Autodesk Inventor part; units mm, degrees
(part 3 of 5)
sketch "Skizze6" plane through (0, 1, 0) normal (0, 1, 0) x (1, 0, 0)
  line L0 (-132.892, -90.8566) -> (-0.05, -90.8566) projected
  line L1 (-0.05, -90.8566) -> (-0.05, -0.0262) projected
  line L2 (-0.05, -0.0262) -> (-132.892, -0.0262) projected
  line L3 (-132.892, -0.0262) -> (-132.892, -90.8566) projected
  line L4 (-22.1876, -19.3868) -> (-20.5876, -19.3868) projected
  line L5 (-20.5876, -19.3868) -> (-20.5876, -20.0368) projected
  line L6 (-20.5876, -20.0368) -> (-22.1876, -20.0368) projected
  line L7 (-22.1876, -20.0368) -> (-22.1876, -19.3868) projected
  line L8 (-22.1876, -11.4868) -> (-20.5876, -11.4868) projected
  line L9 (-20.5876, -11.4868) -> (-20.5876, -12.1368) projected
  line L10 (-20.5876, -12.1368) -> (-22.1876, -12.1368) projected
  line L11 (-22.1876, -12.1368) -> (-22.1876, -11.4868) projected
  line L12 (-23.0526, -18.3618) -> (-22.2626, -18.3618) projected
  line L13 (-22.2626, -18.3618) -> (-22.2626, -18.7618) projected
  line L14 (-22.2626, -18.7618) -> (-23.0526, -18.7618) projected
  line L15 (-23.0526, -18.7618) -> (-23.0526, -18.3618) projected
  line L16 (-20.5126, -18.3618) -> (-19.7226, -18.3618) projected
  line L17 (-19.7226, -18.3618) -> (-19.7226, -18.7618) projected
  line L18 (-19.7226, -18.7618) -> (-20.5126, -18.7618) projected
  line L19 (-20.5126, -18.7618) -> (-20.5126, -18.3618) projected
  line L20 (-23.0526, -17.5618) -> (-22.2626, -17.5618) projected
  line L21 (-22.2626, -17.5618) -> (-22.2626, -17.9618) projected
  line L22 (-22.2626, -17.9618) -> (-23.0526, -17.9618) projected
  line L23 (-23.0526, -17.9618) -> (-23.0526, -17.5618) projected
  line L24 (-20.5126, -17.5618) -> (-19.7226, -17.5618) projected
  line L25 (-19.7226, -17.5618) -> (-19.7226, -17.9618) projected
  line L26 (-19.7226, -17.9618) -> (-20.5126, -17.9618) projected
  line L27 (-20.5126, -17.9618) -> (-20.5126, -17.5618) projected
  line L28 (-23.0526, -16.7618) -> (-22.2626, -16.7618) projected
  line L29 (-22.2626, -16.7618) -> (-22.2626, -17.1618) projected
  line L30 (-22.2626, -17.1618) -> (-23.0526, -17.1618) projected
  line L31 (-23.0526, -17.1618) -> (-23.0526, -16.7618) projected
  line L32 (-20.5126, -16.7618) -> (-19.7226, -16.7618) projected
  line L33 (-19.7226, -16.7618) -> (-19.7226, -17.1618) projected
  line L34 (-19.7226, -17.1618) -> (-20.5126, -17.1618) projected
  line L35 (-20.5126, -17.1618) -> (-20.5126, -16.7618) projected
  line L36 (-23.0526, -15.9618) -> (-22.2626, -15.9618) projected
  line L37 (-22.2626, -15.9618) -> (-22.2626, -16.3618) projected
  line L38 (-22.2626, -16.3618) -> (-23.0526, -16.3618) projected
  line L39 (-23.0526, -16.3618) -> (-23.0526, -15.9618) projected
  line L40 (-20.5126, -15.9618) -> (-19.7226, -15.9618) projected
  line L41 (-19.7226, -15.9618) -> (-19.7226, -16.3618) projected
  line L42 (-19.7226, -16.3618) -> (-20.5126, -16.3618) projected
  line L43 (-20.5126, -16.3618) -> (-20.5126, -15.9618) projected
  line L44 (-23.0526, -15.1618) -> (-22.2626, -15.1618) projected
  line L45 (-22.2626, -15.1618) -> (-22.2626, -15.5618) projected
  line L46 (-22.2626, -15.5618) -> (-23.0526, -15.5618) projected
  line L47 (-23.0526, -15.5618) -> (-23.0526, -15.1618) projected
  line L48 (-20.5126, -15.1618) -> (-19.7226, -15.1618) projected
  line L49 (-19.7226, -15.1618) -> (-19.7226, -15.5618) projected
  line L50 (-19.7226, -15.5618) -> (-20.5126, -15.5618) projected
  line L51 (-20.5126, -15.5618) -> (-20.5126, -15.1618) projected
  line L52 (-23.0526, -14.3618) -> (-22.2626, -14.3618) projected
  line L53 (-22.2626, -14.3618) -> (-22.2626, -14.7618) projected
  line L54 (-22.2626, -14.7618) -> (-23.0526, -14.7618) projected
  line L55 (-23.0526, -14.7618) -> (-23.0526, -14.3618) projected
  line L56 (-20.5126, -14.3618) -> (-19.7226, -14.3618) projected
  line L57 (-19.7226, -14.3618) -> (-19.7226, -14.7618) projected
  line L58 (-19.7226, -14.7618) -> (-20.5126, -14.7618) projected
  line L59 (-20.5126, -14.7618) -> (-20.5126, -14.3618) projected
  line L60 (-23.0526, -13.5618) -> (-22.2626, -13.5618) projected
  line L61 (-22.2626, -13.5618) -> (-22.2626, -13.9618) projected
  line L62 (-22.2626, -13.9618) -> (-23.0526, -13.9618) projected
  line L63 (-23.0526, -13.9618) -> (-23.0526, -13.5618) projected
  line L64 (-20.5126, -13.5618) -> (-19.7226, -13.5618) projected
  line L65 (-19.7226, -13.5618) -> (-19.7226, -13.9618) projected
  line L66 (-19.7226, -13.9618) -> (-20.5126, -13.9618) projected
  line L67 (-20.5126, -13.9618) -> (-20.5126, -13.5618) projected
  line L68 (-23.0526, -12.7618) -> (-22.2626, -12.7618) projected
  line L69 (-22.2626, -12.7618) -> (-22.2626, -13.1618) projected
  line L70 (-22.2626, -13.1618) -> (-23.0526, -13.1618) projected
  line L71 (-23.0526, -13.1618) -> (-23.0526, -12.7618) projected
  line L72 (-20.5126, -12.7618) -> (-19.7226, -12.7618) projected
  line L73 (-19.7226, -12.7618) -> (-19.7226, -13.1618) projected
  line L74 (-19.7226, -13.1618) -> (-20.5126, -13.1618) projected
  line L75 (-20.5126, -13.1618) -> (-20.5126, -12.7618) projected
  line L76 (-95.9651, -30.7118) -> (-97.5651, -30.7118) projected
  line L77 (-97.5651, -30.7118) -> (-97.5651, -30.0618) projected
  line L78 (-97.5651, -30.0618) -> (-95.9651, -30.0618) projected
  line L79 (-95.9651, -30.0618) -> (-95.9651, -30.7118) projected
  line L80 (-95.9651, -38.6118) -> (-97.5651, -38.6118) projected
  line L81 (-97.5651, -38.6118) -> (-97.5651, -37.9618) projected
  line L82 (-97.5651, -37.9618) -> (-95.9651, -37.9618) projected
  line L83 (-95.9651, -37.9618) -> (-95.9651, -38.6118) projected
  line L84 (-95.1001, -31.7368) -> (-95.8901, -31.7368) projected
  line L85 (-95.8901, -31.7368) -> (-95.8901, -31.3368) projected
  line L86 (-95.8901, -31.3368) -> (-95.1001, -31.3368) projected
  line L87 (-95.1001, -31.3368) -> (-95.1001, -31.7368) projected
  line L88 (-97.6401, -31.7368) -> (-98.4301, -31.7368) projected
  line L89 (-98.4301, -31.7368) -> (-98.4301, -31.3368) projected
  line L90 (-98.4301, -31.3368) -> (-97.6401, -31.3368) projected
  line L91 (-97.6401, -31.3368) -> (-97.6401, -31.7368) projected
  line L92 (-95.1001, -32.5368) -> (-95.8901, -32.5368) projected
  line L93 (-95.8901, -32.5368) -> (-95.8901, -32.1368) projected
  line L94 (-95.8901, -32.1368) -> (-95.1001, -32.1368) projected
  line L95 (-95.1001, -32.1368) -> (-95.1001, -32.5368) projected
  line L96 (-97.6401, -32.5368) -> (-98.4301, -32.5368) projected
  line L97 (-98.4301, -32.5368) -> (-98.4301, -32.1368) projected
  line L98 (-98.4301, -32.1368) -> (-97.6401, -32.1368) projected
  line L99 (-97.6401, -32.1368) -> (-97.6401, -32.5368) projected
  line L100 (-95.1001, -33.3368) -> (-95.8901, -33.3368) projected
  line L101 (-95.8901, -33.3368) -> (-95.8901, -32.9368) projected
  line L102 (-95.8901, -32.9368) -> (-95.1001, -32.9368) projected
  line L103 (-95.1001, -32.9368) -> (-95.1001, -33.3368) projected
  line L104 (-97.6401, -33.3368) -> (-98.4301, -33.3368) projected
  line L105 (-98.4301, -33.3368) -> (-98.4301, -32.9368) projected
  line L106 (-98.4301, -32.9368) -> (-97.6401, -32.9368) projected
  line L107 (-97.6401, -32.9368) -> (-97.6401, -33.3368) projected
  line L108 (-95.1001, -34.1368) -> (-95.8901, -34.1368) projected
  line L109 (-95.8901, -34.1368) -> (-95.8901, -33.7368) projected
  line L110 (-95.8901, -33.7368) -> (-95.1001, -33.7368) projected
  line L111 (-95.1001, -33.7368) -> (-95.1001, -34.1368) projected
  line L112 (-97.6401, -34.1368) -> (-98.4301, -34.1368) projected
  line L113 (-98.4301, -34.1368) -> (-98.4301, -33.7368) projected
  line L114 (-98.4301, -33.7368) -> (-97.6401, -33.7368) projected
  line L115 (-97.6401, -33.7368) -> (-97.6401, -34.1368) projected
  line L116 (-95.1001, -34.9368) -> (-95.8901, -34.9368) projected
  line L117 (-95.8901, -34.9368) -> (-95.8901, -34.5368) projected
  line L118 (-95.8901, -34.5368) -> (-95.1001, -34.5368) projected
  line L119 (-95.1001, -34.5368) -> (-95.1001, -34.9368) projected
  line L120 (-97.6401, -34.9368) -> (-98.4301, -34.9368) projected
  line L121 (-98.4301, -34.9368) -> (-98.4301, -34.5368) projected
  line L122 (-98.4301, -34.5368) -> (-97.6401, -34.5368) projected
  line L123 (-97.6401, -34.5368) -> (-97.6401, -34.9368) projected
  line L124 (-95.1001, -35.7368) -> (-95.8901, -35.7368) projected
  line L125 (-95.8901, -35.7368) -> (-95.8901, -35.3368) projected
  line L126 (-95.8901, -35.3368) -> (-95.1001, -35.3368) projected
  line L127 (-95.1001, -35.3368) -> (-95.1001, -35.7368) projected
  line L128 (-97.6401, -35.7368) -> (-98.4301, -35.7368) projected
  line L129 (-98.4301, -35.7368) -> (-98.4301, -35.3368) projected
  line L130 (-98.4301, -35.3368) -> (-97.6401, -35.3368) projected
  line L131 (-97.6401, -35.3368) -> (-97.6401, -35.7368) projected
  line L132 (-95.1001, -36.5368) -> (-95.8901, -36.5368) projected
  line L133 (-95.8901, -36.5368) -> (-95.8901, -36.1368) projected
  line L134 (-95.8901, -36.1368) -> (-95.1001, -36.1368) projected
  line L135 (-95.1001, -36.1368) -> (-95.1001, -36.5368) projected
  line L136 (-97.6401, -36.5368) -> (-98.4301, -36.5368) projected
  line L137 (-98.4301, -36.5368) -> (-98.4301, -36.1368) projected
  line L138 (-98.4301, -36.1368) -> (-97.6401, -36.1368) projected
  line L139 (-97.6401, -36.1368) -> (-97.6401, -36.5368) projected
  line L140 (-95.1001, -37.3368) -> (-95.8901, -37.3368) projected
  line L141 (-95.8901, -37.3368) -> (-95.8901, -36.9368) projected
  line L142 (-95.8901, -36.9368) -> (-95.1001, -36.9368) projected
  line L143 (-95.1001, -36.9368) -> (-95.1001, -37.3368) projected
  line L144 (-97.6401, -37.3368) -> (-98.4301, -37.3368) projected
  line L145 (-98.4301, -37.3368) -> (-98.4301, -36.9368) projected
  line L146 (-98.4301, -36.9368) -> (-97.6401, -36.9368) projected
  line L147 (-97.6401, -36.9368) -> (-97.6401, -37.3368) projected
  line L148 (-77.0826, -68.4118) -> (-78.6826, -68.4118) projected
  line L149 (-78.6826, -68.4118) -> (-78.6826, -67.7618) projected
  line L150 (-78.6826, -67.7618) -> (-77.0826, -67.7618) projected
  line L151 (-77.0826, -67.7618) -> (-77.0826, -68.4118) projected
  line L152 (-77.0826, -76.3118) -> (-78.6826, -76.3118) projected
  line L153 (-78.6826, -76.3118) -> (-78.6826, -75.6618) projected
  line L154 (-78.6826, -75.6618) -> (-77.0826, -75.6618) projected
  line L155 (-77.0826, -75.6618) -> (-77.0826, -76.3118) projected
  line L156 (-76.2176, -69.4368) -> (-77.0076, -69.4368) projected
  line L157 (-77.0076, -69.4368) -> (-77.0076, -69.0368) projected
  line L158 (-77.0076, -69.0368) -> (-76.2176, -69.0368) projected
  line L159 (-76.2176, -69.0368) -> (-76.2176, -69.4368) projected
  line L160 (-78.7576, -69.4368) -> (-79.5476, -69.4368) projected
  line L161 (-79.5476, -69.4368) -> (-79.5476, -69.0368) projected
  line L162 (-79.5476, -69.0368) -> (-78.7576, -69.0368) projected
  line L163 (-78.7576, -69.0368) -> (-78.7576, -69.4368) projected
  line L164 (-76.2176, -70.2368) -> (-77.0076, -70.2368) projected
  line L165 (-77.0076, -70.2368) -> (-77.0076, -69.8368) projected
  line L166 (-77.0076, -69.8368) -> (-76.2176, -69.8368) projected
  line L167 (-76.2176, -69.8368) -> (-76.2176, -70.2368) projected
  line L168 (-78.7576, -70.2368) -> (-79.5476, -70.2368) projected
  line L169 (-79.5476, -70.2368) -> (-79.5476, -69.8368) projected
  line L170 (-79.5476, -69.8368) -> (-78.7576, -69.8368) projected
  line L171 (-78.7576, -69.8368) -> (-78.7576, -70.2368) projected
  line L172 (-76.2176, -71.0368) -> (-77.0076, -71.0368) projected
  line L173 (-77.0076, -71.0368) -> (-77.0076, -70.6368) projected
  line L174 (-77.0076, -70.6368) -> (-76.2176, -70.6368) projected
  line L175 (-76.2176, -70.6368) -> (-76.2176, -71.0368) projected
  line L176 (-78.7576, -71.0368) -> (-79.5476, -71.0368) projected
  line L177 (-79.5476, -71.0368) -> (-79.5476, -70.6368) projected
  line L178 (-79.5476, -70.6368) -> (-78.7576, -70.6368) projected
  line L179 (-78.7576, -70.6368) -> (-78.7576, -71.0368) projected
  line L180 (-76.2176, -71.8368) -> (-77.0076, -71.8368) projected
  line L181 (-77.0076, -71.8368) -> (-77.0076, -71.4368) projected
  line L182 (-77.0076, -71.4368) -> (-76.2176, -71.4368) projected
  line L183 (-76.2176, -71.4368) -> (-76.2176, -71.8368) projected
  line L184 (-78.7576, -71.8368) -> (-79.5476, -71.8368) projected
  line L185 (-79.5476, -71.8368) -> (-79.5476, -71.4368) projected
  line L186 (-79.5476, -71.4368) -> (-78.7576, -71.4368) projected
  line L187 (-78.7576, -71.4368) -> (-78.7576, -71.8368) projected
  line L188 (-76.2176, -72.6368) -> (-77.0076, -72.6368) projected
  line L189 (-77.0076, -72.6368) -> (-77.0076, -72.2368) projected
  line L190 (-77.0076, -72.2368) -> (-76.2176, -72.2368) projected
  line L191 (-76.2176, -72.2368) -> (-76.2176, -72.6368) projected
  line L192 (-78.7576, -72.6368) -> (-79.5476, -72.6368) projected
  line L193 (-79.5476, -72.6368) -> (-79.5476, -72.2368) projected
  line L194 (-79.5476, -72.2368) -> (-78.7576, -72.2368) projected
  line L195 (-78.7576, -72.2368) -> (-78.7576, -72.6368) projected
  line L196 (-76.2176, -73.4368) -> (-77.0076, -73.4368) projected
  line L197 (-77.0076, -73.4368) -> (-77.0076, -73.0368) projected
  line L198 (-77.0076, -73.0368) -> (-76.2176, -73.0368) projected
  line L199 (-76.2176, -73.0368) -> (-76.2176, -73.4368) projected
  line L200 (-78.7576, -73.4368) -> (-79.5476, -73.4368) projected
  line L201 (-79.5476, -73.4368) -> (-79.5476, -73.0368) projected
  line L202 (-79.5476, -73.0368) -> (-78.7576, -73.0368) projected
  line L203 (-78.7576, -73.0368) -> (-78.7576, -73.4368) projected
  line L204 (-76.2176, -74.2368) -> (-77.0076, -74.2368) projected
  line L205 (-77.0076, -74.2368) -> (-77.0076, -73.8368) projected
  line L206 (-77.0076, -73.8368) -> (-76.2176, -73.8368) projected
  line L207 (-76.2176, -73.8368) -> (-76.2176, -74.2368) projected
  line L208 (-78.7576, -74.2368) -> (-79.5476, -74.2368) projected
  line L209 (-79.5476, -74.2368) -> (-79.5476, -73.8368) projected
  line L210 (-79.5476, -73.8368) -> (-78.7576, -73.8368) projected
  line L211 (-78.7576, -73.8368) -> (-78.7576, -74.2368) projected
  line L212 (-76.2176, -75.0368) -> (-77.0076, -75.0368) projected
  line L213 (-77.0076, -75.0368) -> (-77.0076, -74.6368) projected
  line L214 (-77.0076, -74.6368) -> (-76.2176, -74.6368) projected
  line L215 (-76.2176, -74.6368) -> (-76.2176, -75.0368) projected
  line L216 (-78.7576, -75.0368) -> (-79.5476, -75.0368) projected
  line L217 (-79.5476, -75.0368) -> (-79.5476, -74.6368) projected
  line L218 (-79.5476, -74.6368) -> (-78.7576, -74.6368) projected
  line L219 (-78.7576, -74.6368) -> (-78.7576, -75.0368) projected
  line L220 (-58.2826, -30.6368) -> (-59.8826, -30.6368) projected
  line L221 (-59.8826, -30.6368) -> (-59.8826, -29.9868) projected
  line L222 (-59.8826, -29.9868) -> (-58.2826, -29.9868) projected
  line L223 (-58.2826, -29.9868) -> (-58.2826, -30.6368) projected
  line L224 (-58.2826, -38.5368) -> (-59.8826, -38.5368) projected
  line L225 (-59.8826, -38.5368) -> (-59.8826, -37.8868) projected
  line L226 (-59.8826, -37.8868) -> (-58.2826, -37.8868) projected
  line L227 (-58.2826, -37.8868) -> (-58.2826, -38.5368) projected
  line L228 (-57.4176, -31.6618) -> (-58.2076, -31.6618) projected
  line L229 (-58.2076, -31.6618) -> (-58.2076, -31.2618) projected
  line L230 (-58.2076, -31.2618) -> (-57.4176, -31.2618) projected
  line L231 (-57.4176, -31.2618) -> (-57.4176, -31.6618) projected
  line L232 (-59.9576, -31.6618) -> (-60.7476, -31.6618) projected
  line L233 (-60.7476, -31.6618) -> (-60.7476, -31.2618) projected
  line L234 (-60.7476, -31.2618) -> (-59.9576, -31.2618) projected
  line L235 (-59.9576, -31.2618) -> (-59.9576, -31.6618) projected
  line L236 (-57.4176, -32.4618) -> (-58.2076, -32.4618) projected
  line L237 (-58.2076, -32.4618) -> (-58.2076, -32.0618) projected
  line L238 (-58.2076, -32.0618) -> (-57.4176, -32.0618) projected
  line L239 (-57.4176, -32.0618) -> (-57.4176, -32.4618) projected
  line L240 (-59.9576, -32.4618) -> (-60.7476, -32.4618) projected
  line L241 (-60.7476, -32.4618) -> (-60.7476, -32.0618) projected
  line L242 (-60.7476, -32.0618) -> (-59.9576, -32.0618) projected
  line L243 (-59.9576, -32.0618) -> (-59.9576, -32.4618) projected
  line L244 (-57.4176, -33.2618) -> (-58.2076, -33.2618) projected
  line L245 (-58.2076, -33.2618) -> (-58.2076, -32.8618) projected
  line L246 (-58.2076, -32.8618) -> (-57.4176, -32.8618) projected
  line L247 (-57.4176, -32.8618) -> (-57.4176, -33.2618) projected
  line L248 (-59.9576, -33.2618) -> (-60.7476, -33.2618) projected
  line L249 (-60.7476, -33.2618) -> (-60.7476, -32.8618) projected
  line L250 (-60.7476, -32.8618) -> (-59.9576, -32.8618) projected
  line L251 (-59.9576, -32.8618) -> (-59.9576, -33.2618) projected
  line L252 (-57.4176, -34.0618) -> (-58.2076, -34.0618) projected
  line L253 (-58.2076, -34.0618) -> (-58.2076, -33.6618) projected
  line L254 (-58.2076, -33.6618) -> (-57.4176, -33.6618) projected
  line L255 (-57.4176, -33.6618) -> (-57.4176, -34.0618) projected
  line L256 (-59.9576, -34.0618) -> (-60.7476, -34.0618) projected
  line L257 (-60.7476, -34.0618) -> (-60.7476, -33.6618) projected
  line L258 (-60.7476, -33.6618) -> (-59.9576, -33.6618) projected
  line L259 (-59.9576, -33.6618) -> (-59.9576, -34.0618) projected
  line L260 (-57.4176, -34.8618) -> (-58.2076, -34.8618) projected
  line L261 (-58.2076, -34.8618) -> (-58.2076, -34.4618) projected
  line L262 (-58.2076, -34.4618) -> (-57.4176, -34.4618) projected
  line L263 (-57.4176, -34.4618) -> (-57.4176, -34.8618) projected
  line L264 (-59.9576, -34.8618) -> (-60.7476, -34.8618) projected
  line L265 (-60.7476, -34.8618) -> (-60.7476, -34.4618) projected
  line L266 (-60.7476, -34.4618) -> (-59.9576, -34.4618) projected
  line L267 (-59.9576, -34.4618) -> (-59.9576, -34.8618) projected
  line L268 (-57.4176, -35.6618) -> (-58.2076, -35.6618) projected
  line L269 (-58.2076, -35.6618) -> (-58.2076, -35.2618) projected
  line L270 (-58.2076, -35.2618) -> (-57.4176, -35.2618) projected
  line L271 (-57.4176, -35.2618) -> (-57.4176, -35.6618) projected
  line L272 (-59.9576, -35.6618) -> (-60.7476, -35.6618) projected
  line L273 (-60.7476, -35.6618) -> (-60.7476, -35.2618) projected
  line L274 (-60.7476, -35.2618) -> (-59.9576, -35.2618) projected
  line L275 (-59.9576, -35.2618) -> (-59.9576, -35.6618) projected
  line L276 (-57.4176, -36.4618) -> (-58.2076, -36.4618) projected
  line L277 (-58.2076, -36.4618) -> (-58.2076, -36.0618) projected
  line L278 (-58.2076, -36.0618) -> (-57.4176, -36.0618) projected
  line L279 (-57.4176, -36.0618) -> (-57.4176, -36.4618) projected
  line L280 (-59.9576, -36.4618) -> (-60.7476, -36.4618) projected
  line L281 (-60.7476, -36.4618) -> (-60.7476, -36.0618) projected
  line L282 (-60.7476, -36.0618) -> (-59.9576, -36.0618) projected
  line L283 (-59.9576, -36.0618) -> (-59.9576, -36.4618) projected
  line L284 (-57.4176, -37.2618) -> (-58.2076, -37.2618) projected
  line L285 (-58.2076, -37.2618) -> (-58.2076, -36.8618) projected
  line L286 (-58.2076, -36.8618) -> (-57.4176, -36.8618) projected
  line L287 (-57.4176, -36.8618) -> (-57.4176, -37.2618) projected
  line L288 (-59.9576, -37.2618) -> (-60.7476, -37.2618) projected
  line L289 (-60.7476, -37.2618) -> (-60.7476, -36.8618) projected
  line L290 (-60.7476, -36.8618) -> (-59.9576, -36.8618) projected
  line L291 (-59.9576, -36.8618) -> (-59.9576, -37.2618) projected
  line L292 (-22.0301, -57.0618) -> (-20.4301, -57.0618) projected
  line L293 (-20.4301, -57.0618) -> (-20.4301, -57.7118) projected
  line L294 (-20.4301, -57.7118) -> (-22.0301, -57.7118) projected
  line L295 (-22.0301, -57.7118) -> (-22.0301, -57.0618) projected
  line L296 (-22.0301, -49.1618) -> (-20.4301, -49.1618) projected
  line L297 (-20.4301, -49.1618) -> (-20.4301, -49.8118) projected
  line L298 (-20.4301, -49.8118) -> (-22.0301, -49.8118) projected
  line L299 (-22.0301, -49.8118) -> (-22.0301, -49.1618) projected
  line L300 (-22.8951, -56.0368) -> (-22.1051, -56.0368) projected
  line L301 (-22.1051, -56.0368) -> (-22.1051, -56.4368) projected
  line L302 (-22.1051, -56.4368) -> (-22.8951, -56.4368) projected
  line L303 (-22.8951, -56.4368) -> (-22.8951, -56.0368) projected
  line L304 (-20.3551, -56.0368) -> (-19.5651, -56.0368) projected
  line L305 (-19.5651, -56.0368) -> (-19.5651, -56.4368) projected
  line L306 (-19.5651, -56.4368) -> (-20.3551, -56.4368) projected
  line L307 (-20.3551, -56.4368) -> (-20.3551, -56.0368) projected
  line L308 (-22.8951, -55.2368) -> (-22.1051, -55.2368) projected
  line L309 (-22.1051, -55.2368) -> (-22.1051, -55.6368) projected
  line L310 (-22.1051, -55.6368) -> (-22.8951, -55.6368) projected
  line L311 (-22.8951, -55.6368) -> (-22.8951, -55.2368) projected
  line L312 (-20.3551, -55.2368) -> (-19.5651, -55.2368) projected
  line L313 (-19.5651, -55.2368) -> (-19.5651, -55.6368) projected
  line L314 (-19.5651, -55.6368) -> (-20.3551, -55.6368) projected
  line L315 (-20.3551, -55.6368) -> (-20.3551, -55.2368) projected
  line L316 (-22.8951, -54.4368) -> (-22.1051, -54.4368) projected
  line L317 (-22.1051, -54.4368) -> (-22.1051, -54.8368) projected
  line L318 (-22.1051, -54.8368) -> (-22.8951, -54.8368) projected
  line L319 (-22.8951, -54.8368) -> (-22.8951, -54.4368) projected
  line L320 (-20.3551, -54.4368) -> (-19.5651, -54.4368) projected
  line L321 (-19.5651, -54.4368) -> (-19.5651, -54.8368) projected
  line L322 (-19.5651, -54.8368) -> (-20.3551, -54.8368) projected
  line L323 (-20.3551, -54.8368) -> (-20.3551, -54.4368) projected
  line L324 (-22.8951, -53.6368) -> (-22.1051, -53.6368) projected
  line L325 (-22.1051, -53.6368) -> (-22.1051, -54.0368) projected
  line L326 (-22.1051, -54.0368) -> (-22.8951, -54.0368) projected
  line L327 (-22.8951, -54.0368) -> (-22.8951, -53.6368) projected
  line L328 (-20.3551, -53.6368) -> (-19.5651, -53.6368) projected
  line L329 (-19.5651, -53.6368) -> (-19.5651, -54.0368) projected
  line L330 (-19.5651, -54.0368) -> (-20.3551, -54.0368) projected
  line L331 (-20.3551, -54.0368) -> (-20.3551, -53.6368) projected
  line L332 (-22.8951, -52.8368) -> (-22.1051, -52.8368) projected
  line L333 (-22.1051, -52.8368) -> (-22.1051, -53.2368) projected
  line L334 (-22.1051, -53.2368) -> (-22.8951, -53.2368) projected
  line L335 (-22.8951, -53.2368) -> (-22.8951, -52.8368) projected
  line L336 (-20.3551, -52.8368) -> (-19.5651, -52.8368) projected
  line L337 (-19.5651, -52.8368) -> (-19.5651, -53.2368) projected
  line L338 (-19.5651, -53.2368) -> (-20.3551, -53.2368) projected
  line L339 (-20.3551, -53.2368) -> (-20.3551, -52.8368) projected
  line L340 (-22.8951, -52.0368) -> (-22.1051, -52.0368) projected
  line L341 (-22.1051, -52.0368) -> (-22.1051, -52.4368) projected
  line L342 (-22.1051, -52.4368) -> (-22.8951, -52.4368) projected
  line L343 (-22.8951, -52.4368) -> (-22.8951, -52.0368) projected
  line L344 (-20.3551, -52.0368) -> (-19.5651, -52.0368) projected
  line L345 (-19.5651, -52.0368) -> (-19.5651, -52.4368) projected
  line L346 (-19.5651, -52.4368) -> (-20.3551, -52.4368) projected
  line L347 (-20.3551, -52.4368) -> (-20.3551, -52.0368) projected
  line L348 (-22.8951, -51.2368) -> (-22.1051, -51.2368) projected
  line L349 (-22.1051, -51.2368) -> (-22.1051, -51.6368) projected
  line L350 (-22.1051, -51.6368) -> (-22.8951, -51.6368) projected
  line L351 (-22.8951, -51.6368) -> (-22.8951, -51.2368) projected
  line L352 (-20.3551, -51.2368) -> (-19.5651, -51.2368) projected
  line L353 (-19.5651, -51.2368) -> (-19.5651, -51.6368) projected
  line L354 (-19.5651, -51.6368) -> (-20.3551, -51.6368) projected
  line L355 (-20.3551, -51.6368) -> (-20.3551, -51.2368) projected
  line L356 (-22.8951, -50.4368) -> (-22.1051, -50.4368) projected
  line L357 (-22.1051, -50.4368) -> (-22.1051, -50.8368) projected
  line L358 (-22.1051, -50.8368) -> (-22.8951, -50.8368) projected
  line L359 (-22.8951, -50.8368) -> (-22.8951, -50.4368) projected
  line L360 (-20.3551, -50.4368) -> (-19.5651, -50.4368) projected
  line L361 (-19.5651, -50.4368) -> (-19.5651, -50.8368) projected
  line L362 (-19.5651, -50.8368) -> (-20.3551, -50.8368) projected
  line L363 (-20.3551, -50.8368) -> (-20.3551, -50.4368) projected
  line L364 (-39.3826, -68.5118) -> (-40.9826, -68.5118) projected
  line L365 (-40.9826, -68.5118) -> (-40.9826, -67.8618) projected
  line L366 (-40.9826, -67.8618) -> (-39.3826, -67.8618) projected
  line L367 (-39.3826, -67.8618) -> (-39.3826, -68.5118) projected
  line L368 (-39.3826, -76.4118) -> (-40.9826, -76.4118) projected
  line L369 (-40.9826, -76.4118) -> (-40.9826, -75.7618) projected
  line L370 (-40.9826, -75.7618) -> (-39.3826, -75.7618) projected
  line L371 (-39.3826, -75.7618) -> (-39.3826, -76.4118) projected
  line L372 (-38.5176, -69.5368) -> (-39.3076, -69.5368) projected
  line L373 (-39.3076, -69.5368) -> (-39.3076, -69.1368) projected
  line L374 (-39.3076, -69.1368) -> (-38.5176, -69.1368) projected
  line L375 (-38.5176, -69.1368) -> (-38.5176, -69.5368) projected
  line L376 (-41.0576, -69.5368) -> (-41.8476, -69.5368) projected
  line L377 (-41.8476, -69.5368) -> (-41.8476, -69.1368) projected
  line L378 (-41.8476, -69.1368) -> (-41.0576, -69.1368) projected
  line L379 (-41.0576, -69.1368) -> (-41.0576, -69.5368) projected
  line L380 (-38.5176, -70.3368) -> (-39.3076, -70.3368) projected
  line L381 (-39.3076, -70.3368) -> (-39.3076, -69.9368) projected
  line L382 (-39.3076, -69.9368) -> (-38.5176, -69.9368) projected
  line L383 (-38.5176, -69.9368) -> (-38.5176, -70.3368) projected
  line L384 (-41.0576, -70.3368) -> (-41.8476, -70.3368) projected
  line L385 (-41.8476, -70.3368) -> (-41.8476, -69.9368) projected
  line L386 (-41.8476, -69.9368) -> (-41.0576, -69.9368) projected
  line L387 (-41.0576, -69.9368) -> (-41.0576, -70.3368) projected
  line L388 (-38.5176, -71.1368) -> (-39.3076, -71.1368) projected
  line L389 (-39.3076, -71.1368) -> (-39.3076, -70.7368) projected
  line L390 (-39.3076, -70.7368) -> (-38.5176, -70.7368) projected
  line L391 (-38.5176, -70.7368) -> (-38.5176, -71.1368) projected
  line L392 (-41.0576, -71.1368) -> (-41.8476, -71.1368) projected
  line L393 (-41.8476, -71.1368) -> (-41.8476, -70.7368) projected
  line L394 (-41.8476, -70.7368) -> (-41.0576, -70.7368) projected
  line L395 (-41.0576, -70.7368) -> (-41.0576, -71.1368) projected
  line L396 (-38.5176, -71.9368) -> (-39.3076, -71.9368) projected
  line L397 (-39.3076, -71.9368) -> (-39.3076, -71.5368) projected
  line L398 (-39.3076, -71.5368) -> (-38.5176, -71.5368) projected
  line L399 (-38.5176, -71.5368) -> (-38.5176, -71.9368) projected
  line L400 (-41.0576, -71.9368) -> (-41.8476, -71.9368) projected
  line L401 (-41.8476, -71.9368) -> (-41.8476, -71.5368) projected
  line L402 (-41.8476, -71.5368) -> (-41.0576, -71.5368) projected
  line L403 (-41.0576, -71.5368) -> (-41.0576, -71.9368) projected
  line L404 (-38.5176, -72.7368) -> (-39.3076, -72.7368) projected
  line L405 (-39.3076, -72.7368) -> (-39.3076, -72.3368) projected
  line L406 (-39.3076, -72.3368) -> (-38.5176, -72.3368) projected
  line L407 (-38.5176, -72.3368) -> (-38.5176, -72.7368) projected
  line L408 (-41.0576, -72.7368) -> (-41.8476, -72.7368) projected
  line L409 (-41.8476, -72.7368) -> (-41.8476, -72.3368) projected
  line L410 (-41.8476, -72.3368) -> (-41.0576, -72.3368) projected
  line L411 (-41.0576, -72.3368) -> (-41.0576, -72.7368) projected
  line L412 (-38.5176, -73.5368) -> (-39.3076, -73.5368) projected
  line L413 (-39.3076, -73.5368) -> (-39.3076, -73.1368) projected
  line L414 (-39.3076, -73.1368) -> (-38.5176, -73.1368) projected
  line L415 (-38.5176, -73.1368) -> (-38.5176, -73.5368) projected
  line L416 (-41.0576, -73.5368) -> (-41.8476, -73.5368) projected
  line L417 (-41.8476, -73.5368) -> (-41.8476, -73.1368) projected
  line L418 (-41.8476, -73.1368) -> (-41.0576, -73.1368) projected
  line L419 (-41.0576, -73.1368) -> (-41.0576, -73.5368) projected
  line L420 (-38.5176, -74.3368) -> (-39.3076, -74.3368) projected
  line L421 (-39.3076, -74.3368) -> (-39.3076, -73.9368) projected
  line L422 (-39.3076, -73.9368) -> (-38.5176, -73.9368) projected
  line L423 (-38.5176, -73.9368) -> (-38.5176, -74.3368) projected
  line L424 (-41.0576, -74.3368) -> (-41.8476, -74.3368) projected
  line L425 (-41.8476, -74.3368) -> (-41.8476, -73.9368) projected
  line L426 (-41.8476, -73.9368) -> (-41.0576, -73.9368) projected
  line L427 (-41.0576, -73.9368) -> (-41.0576, -74.3368) projected
  line L428 (-38.5176, -75.1368) -> (-39.3076, -75.1368) projected
  line L429 (-39.3076, -75.1368) -> (-39.3076, -74.7368) projected
  line L430 (-39.3076, -74.7368) -> (-38.5176, -74.7368) projected
  line L431 (-38.5176, -74.7368) -> (-38.5176, -75.1368) projected
  line L432 (-41.0576, -75.1368) -> (-41.8476, -75.1368) projected
  line L433 (-41.8476, -75.1368) -> (-41.8476, -74.7368) projected
  line L434 (-41.8476, -74.7368) -> (-41.0576, -74.7368) projected
  line L435 (-41.0576, -74.7368) -> (-41.0576, -75.1368) projected
  line L436 (-59.5926, -57.1118) -> (-57.9926, -57.1118) projected
  line L437 (-57.9926, -57.1118) -> (-57.9926, -57.7618) projected
  line L438 (-57.9926, -57.7618) -> (-59.5926, -57.7618) projected
  line L439 (-59.5926, -57.7618) -> (-59.5926, -57.1118) projected
  line L440 (-59.5926, -49.2118) -> (-57.9926, -49.2118) projected
  line L441 (-57.9926, -49.2118) -> (-57.9926, -49.8618) projected
  line L442 (-57.9926, -49.8618) -> (-59.5926, -49.8618) projected
  line L443 (-59.5926, -49.8618) -> (-59.5926, -49.2118) projected
  line L444 (-60.4576, -56.0868) -> (-59.6676, -56.0868) projected
  line L445 (-59.6676, -56.0868) -> (-59.6676, -56.4868) projected
  line L446 (-59.6676, -56.4868) -> (-60.4576, -56.4868) projected
  line L447 (-60.4576, -56.4868) -> (-60.4576, -56.0868) projected
  line L448 (-57.9176, -56.0868) -> (-57.1276, -56.0868) projected
  line L449 (-57.1276, -56.0868) -> (-57.1276, -56.4868) projected
  line L450 (-57.1276, -56.4868) -> (-57.9176, -56.4868) projected
  line L451 (-57.9176, -56.4868) -> (-57.9176, -56.0868) projected
  line L452 (-60.4576, -55.2868) -> (-59.6676, -55.2868) projected
  line L453 (-59.6676, -55.2868) -> (-59.6676, -55.6868) projected
  line L454 (-59.6676, -55.6868) -> (-60.4576, -55.6868) projected
  line L455 (-60.4576, -55.6868) -> (-60.4576, -55.2868) projected
  line L456 (-57.9176, -55.2868) -> (-57.1276, -55.2868) projected
  line L457 (-57.1276, -55.2868) -> (-57.1276, -55.6868) projected
  line L458 (-57.1276, -55.6868) -> (-57.9176, -55.6868) projected
  line L459 (-57.9176, -55.6868) -> (-57.9176, -55.2868) projected
  line L460 (-60.4576, -54.4868) -> (-59.6676, -54.4868) projected
  line L461 (-59.6676, -54.4868) -> (-59.6676, -54.8868) projected
  line L462 (-59.6676, -54.8868) -> (-60.4576, -54.8868) projected
  line L463 (-60.4576, -54.8868) -> (-60.4576, -54.4868) projected
  line L464 (-57.9176, -54.4868) -> (-57.1276, -54.4868) projected
  line L465 (-57.1276, -54.4868) -> (-57.1276, -54.8868) projected
  line L466 (-57.1276, -54.8868) -> (-57.9176, -54.8868) projected
  line L467 (-57.9176, -54.8868) -> (-57.9176, -54.4868) projected
  line L468 (-60.4576, -53.6868) -> (-59.6676, -53.6868) projected
  line L469 (-59.6676, -53.6868) -> (-59.6676, -54.0868) projected
  line L470 (-59.6676, -54.0868) -> (-60.4576, -54.0868) projected
  line L471 (-60.4576, -54.0868) -> (-60.4576, -53.6868) projected
  line L472 (-57.9176, -53.6868) -> (-57.1276, -53.6868) projected
  line L473 (-57.1276, -53.6868) -> (-57.1276, -54.0868) projected
  line L474 (-57.1276, -54.0868) -> (-57.9176, -54.0868) projected
  line L475 (-57.9176, -54.0868) -> (-57.9176, -53.6868) projected
  line L476 (-60.4576, -52.8868) -> (-59.6676, -52.8868) projected
  line L477 (-59.6676, -52.8868) -> (-59.6676, -53.2868) projected
  line L478 (-59.6676, -53.2868) -> (-60.4576, -53.2868) projected
  line L479 (-60.4576, -53.2868) -> (-60.4576, -52.8868) projected
  line L480 (-57.9176, -52.8868) -> (-57.1276, -52.8868) projected
  line L481 (-57.1276, -52.8868) -> (-57.1276, -53.2868) projected
  line L482 (-57.1276, -53.2868) -> (-57.9176, -53.2868) projected
  line L483 (-57.9176, -53.2868) -> (-57.9176, -52.8868) projected
  line L484 (-60.4576, -52.0868) -> (-59.6676, -52.0868) projected
  line L485 (-59.6676, -52.0868) -> (-59.6676, -52.4868) projected
  line L486 (-59.6676, -52.4868) -> (-60.4576, -52.4868) projected
  line L487 (-60.4576, -52.4868) -> (-60.4576, -52.0868) projected
  line L488 (-57.9176, -52.0868) -> (-57.1276, -52.0868) projected
  line L489 (-57.1276, -52.0868) -> (-57.1276, -52.4868) projected
  line L490 (-57.1276, -52.4868) -> (-57.9176, -52.4868) projected
  line L491 (-57.9176, -52.4868) -> (-57.9176, -52.0868) projected
  line L492 (-60.4576, -51.2868) -> (-59.6676, -51.2868) projected
  line L493 (-59.6676, -51.2868) -> (-59.6676, -51.6868) projected
  line L494 (-59.6676, -51.6868) -> (-60.4576, -51.6868) projected
  line L495 (-60.4576, -51.6868) -> (-60.4576, -51.2868) projected
  line L496 (-57.9176, -51.2868) -> (-57.1276, -51.2868) projected
  line L497 (-57.1276, -51.2868) -> (-57.1276, -51.6868) projected
  line L498 (-57.1276, -51.6868) -> (-57.9176, -51.6868) projected
  line L499 (-57.9176, -51.6868) -> (-57.9176, -51.2868) projected
  line L500 (-60.4576, -50.4868) -> (-59.6676, -50.4868) projected
  line L501 (-59.6676, -50.4868) -> (-59.6676, -50.8868) projected
  line L502 (-59.6676, -50.8868) -> (-60.4576, -50.8868) projected
  line L503 (-60.4576, -50.8868) -> (-60.4576, -50.4868) projected
  line L504 (-57.9176, -50.4868) -> (-57.1276, -50.4868) projected
  line L505 (-57.1276, -50.4868) -> (-57.1276, -50.8868) projected
  line L506 (-57.1276, -50.8868) -> (-57.9176, -50.8868) projected
  line L507 (-57.9176, -50.8868) -> (-57.9176, -50.4868) projected
  line L508 (-116.3426, -56.9868) -> (-114.7426, -56.9868) projected
  line L509 (-114.7426, -56.9868) -> (-114.7426, -57.6368) projected
  line L510 (-114.7426, -57.6368) -> (-116.3426, -57.6368) projected
  line L511 (-116.3426, -57.6368) -> (-116.3426, -56.9868) projected
  line L512 (-116.3426, -49.0868) -> (-114.7426, -49.0868) projected
  line L513 (-114.7426, -49.0868) -> (-114.7426, -49.7368) projected
  line L514 (-114.7426, -49.7368) -> (-116.3426, -49.7368) projected
  line L515 (-116.3426, -49.7368) -> (-116.3426, -49.0868) projected
  line L516 (-117.2076, -55.9618) -> (-116.4176, -55.9618) projected
  line L517 (-116.4176, -55.9618) -> (-116.4176, -56.3618) projected
  line L518 (-116.4176, -56.3618) -> (-117.2076, -56.3618) projected
  line L519 (-117.2076, -56.3618) -> (-117.2076, -55.9618) projected
  line L520 (-114.6676, -55.9618) -> (-113.8776, -55.9618) projected
  line L521 (-113.8776, -55.9618) -> (-113.8776, -56.3618) projected
  line L522 (-113.8776, -56.3618) -> (-114.6676, -56.3618) projected
  line L523 (-114.6676, -56.3618) -> (-114.6676, -55.9618) projected
  line L524 (-117.2076, -55.1618) -> (-116.4176, -55.1618) projected
  line L525 (-116.4176, -55.1618) -> (-116.4176, -55.5618) projected
  line L526 (-116.4176, -55.5618) -> (-117.2076, -55.5618) projected
  line L527 (-117.2076, -55.5618) -> (-117.2076, -55.1618) projected
  line L528 (-114.6676, -55.1618) -> (-113.8776, -55.1618) projected
  line L529 (-113.8776, -55.1618) -> (-113.8776, -55.5618) projected
  line L530 (-113.8776, -55.5618) -> (-114.6676, -55.5618) projected
  line L531 (-114.6676, -55.5618) -> (-114.6676, -55.1618) projected
  line L532 (-117.2076, -54.3618) -> (-116.4176, -54.3618) projected
  line L533 (-116.4176, -54.3618) -> (-116.4176, -54.7618) projected
  line L534 (-116.4176, -54.7618) -> (-117.2076, -54.7618) projected
  line L535 (-117.2076, -54.7618) -> (-117.2076, -54.3618) projected
  line L536 (-114.6676, -54.3618) -> (-113.8776, -54.3618) projected
  line L537 (-113.8776, -54.3618) -> (-113.8776, -54.7618) projected
  line L538 (-113.8776, -54.7618) -> (-114.6676, -54.7618) projected
  line L539 (-114.6676, -54.7618) -> (-114.6676, -54.3618) projected
  line L540 (-117.2076, -53.5618) -> (-116.4176, -53.5618) projected
  line L541 (-116.4176, -53.5618) -> (-116.4176, -53.9618) projected
  line L542 (-116.4176, -53.9618) -> (-117.2076, -53.9618) projected
  line L543 (-117.2076, -53.9618) -> (-117.2076, -53.5618) projected
  line L544 (-114.6676, -53.5618) -> (-113.8776, -53.5618) projected
  line L545 (-113.8776, -53.5618) -> (-113.8776, -53.9618) projected
  line L546 (-113.8776, -53.9618) -> (-114.6676, -53.9618) projected
  line L547 (-114.6676, -53.9618) -> (-114.6676, -53.5618) projected
  line L548 (-117.2076, -52.7618) -> (-116.4176, -52.7618) projected
  line L549 (-116.4176, -52.7618) -> (-116.4176, -53.1618) projected
  line L550 (-116.4176, -53.1618) -> (-117.2076, -53.1618) projected
  line L551 (-117.2076, -53.1618) -> (-117.2076, -52.7618) projected
  line L552 (-114.6676, -52.7618) -> (-113.8776, -52.7618) projected
  line L553 (-113.8776, -52.7618) -> (-113.8776, -53.1618) projected
  line L554 (-113.8776, -53.1618) -> (-114.6676, -53.1618) projected
  line L555 (-114.6676, -53.1618) -> (-114.6676, -52.7618) projected
  line L556 (-117.2076, -51.9618) -> (-116.4176, -51.9618) projected
  line L557 (-116.4176, -51.9618) -> (-116.4176, -52.3618) projected
  line L558 (-116.4176, -52.3618) -> (-117.2076, -52.3618) projected
  line L559 (-117.2076, -52.3618) -> (-117.2076, -51.9618) projected
  line L560 (-114.6676, -51.9618) -> (-113.8776, -51.9618) projected
  line L561 (-113.8776, -51.9618) -> (-113.8776, -52.3618) projected
  line L562 (-113.8776, -52.3618) -> (-114.6676, -52.3618) projected
  line L563 (-114.6676, -52.3618) -> (-114.6676, -51.9618) projected
  line L564 (-117.2076, -51.1618) -> (-116.4176, -51.1618) projected
  line L565 (-116.4176, -51.1618) -> (-116.4176, -51.5618) projected
  line L566 (-116.4176, -51.5618) -> (-117.2076, -51.5618) projected
  line L567 (-117.2076, -51.5618) -> (-117.2076, -51.1618) projected
  line L568 (-114.6676, -51.1618) -> (-113.8776, -51.1618) projected
  line L569 (-113.8776, -51.1618) -> (-113.8776, -51.5618) projected
  line L570 (-113.8776, -51.5618) -> (-114.6676, -51.5618) projected
  line L571 (-114.6676, -51.5618) -> (-114.6676, -51.1618) projected
  line L572 (-117.2076, -50.3618) -> (-116.4176, -50.3618) projected
  line L573 (-116.4176, -50.3618) -> (-116.4176, -50.7618) projected
  line L574 (-116.4176, -50.7618) -> (-117.2076, -50.7618) projected
  line L575 (-117.2076, -50.7618) -> (-117.2076, -50.3618) projected
  line L576 (-114.6676, -50.3618) -> (-113.8776, -50.3618) projected
  line L577 (-113.8776, -50.3618) -> (-113.8776, -50.7618) projected
  line L578 (-113.8776, -50.7618) -> (-114.6676, -50.7618) projected
  line L579 (-114.6676, -50.7618) -> (-114.6676, -50.3618) projected
  line L580 (-95.8901, -68.4868) -> (-97.4901, -68.4868) projected
  line L581 (-97.4901, -68.4868) -> (-97.4901, -67.8368) projected
  line L582 (-97.4901, -67.8368) -> (-95.8901, -67.8368) projected
  line L583 (-95.8901, -67.8368) -> (-95.8901, -68.4868) projected
  line L584 (-95.8901, -76.3868) -> (-97.4901, -76.3868) projected
  line L585 (-97.4901, -76.3868) -> (-97.4901, -75.7368) projected
  line L586 (-97.4901, -75.7368) -> (-95.8901, -75.7368) projected
  line L587 (-95.8901, -75.7368) -> (-95.8901, -76.3868) projected
  line L588 (-95.0251, -69.5118) -> (-95.8151, -69.5118) projected
  line L589 (-95.8151, -69.5118) -> (-95.8151, -69.1118) projected
  line L590 (-95.8151, -69.1118) -> (-95.0251, -69.1118) projected
  line L591 (-95.0251, -69.1118) -> (-95.0251, -69.5118) projected
  line L592 (-97.5651, -69.5118) -> (-98.3551, -69.5118) projected
  line L593 (-98.3551, -69.5118) -> (-98.3551, -69.1118) projected
  line L594 (-98.3551, -69.1118) -> (-97.5651, -69.1118) projected
  line L595 (-97.5651, -69.1118) -> (-97.5651, -69.5118) projected
  line L596 (-95.0251, -70.3118) -> (-95.8151, -70.3118) projected
  line L597 (-95.8151, -70.3118) -> (-95.8151, -69.9118) projected
  line L598 (-95.8151, -69.9118) -> (-95.0251, -69.9118) projected
  line L599 (-95.0251, -69.9118) -> (-95.0251, -70.3118) projected
  line L600 (-97.5651, -70.3118) -> (-98.3551, -70.3118) projected
  line L601 (-98.3551, -70.3118) -> (-98.3551, -69.9118) projected
  line L602 (-98.3551, -69.9118) -> (-97.5651, -69.9118) projected
  line L603 (-97.5651, -69.9118) -> (-97.5651, -70.3118) projected
  line L604 (-95.0251, -71.1118) -> (-95.8151, -71.1118) projected
  line L605 (-95.8151, -71.1118) -> (-95.8151, -70.7118) projected
  line L606 (-95.8151, -70.7118) -> (-95.0251, -70.7118) projected
  line L607 (-95.0251, -70.7118) -> (-95.0251, -71.1118) projected
  line L608 (-97.5651, -71.1118) -> (-98.3551, -71.1118) projected
  line L609 (-98.3551, -71.1118) -> (-98.3551, -70.7118) projected
  line L610 (-98.3551, -70.7118) -> (-97.5651, -70.7118) projected
  line L611 (-97.5651, -70.7118) -> (-97.5651, -71.1118) projected
  line L612 (-95.0251, -71.9118) -> (-95.8151, -71.9118) projected
  line L613 (-95.8151, -71.9118) -> (-95.8151, -71.5118) projected
  line L614 (-95.8151, -71.5118) -> (-95.0251, -71.5118) projected
  line L615 (-95.0251, -71.5118) -> (-95.0251, -71.9118) projected
  line L616 (-97.5651, -71.9118) -> (-98.3551, -71.9118) projected
  line L617 (-98.3551, -71.9118) -> (-98.3551, -71.5118) projected
  line L618 (-98.3551, -71.5118) -> (-97.5651, -71.5118) projected
  line L619 (-97.5651, -71.5118) -> (-97.5651, -71.9118) projected
  line L620 (-95.0251, -72.7118) -> (-95.8151, -72.7118) projected
  line L621 (-95.8151, -72.7118) -> (-95.8151, -72.3118) projected
  line L622 (-95.8151, -72.3118) -> (-95.0251, -72.3118) projected
  line L623 (-95.0251, -72.3118) -> (-95.0251, -72.7118) projected
  line L624 (-97.5651, -72.7118) -> (-98.3551, -72.7118) projected
  line L625 (-98.3551, -72.7118) -> (-98.3551, -72.3118) projected
  line L626 (-98.3551, -72.3118) -> (-97.5651, -72.3118) projected
  line L627 (-97.5651, -72.3118) -> (-97.5651, -72.7118) projected
  line L628 (-95.0251, -73.5118) -> (-95.8151, -73.5118) projected
  line L629 (-95.8151, -73.5118) -> (-95.8151, -73.1118) projected
  line L630 (-95.8151, -73.1118) -> (-95.0251, -73.1118) projected
  line L631 (-95.0251, -73.1118) -> (-95.0251, -73.5118) projected
  line L632 (-97.5651, -73.5118) -> (-98.3551, -73.5118) projected
  line L633 (-98.3551, -73.5118) -> (-98.3551, -73.1118) projected
  line L634 (-98.3551, -73.1118) -> (-97.5651, -73.1118) projected
  line L635 (-97.5651, -73.1118) -> (-97.5651, -73.5118) projected
  line L636 (-95.0251, -74.3118) -> (-95.8151, -74.3118) projected
  line L637 (-95.8151, -74.3118) -> (-95.8151, -73.9118) projected
  line L638 (-95.8151, -73.9118) -> (-95.0251, -73.9118) projected
  line L639 (-95.0251, -73.9118) -> (-95.0251, -74.3118) projected
  line L640 (-97.5651, -74.3118) -> (-98.3551, -74.3118) projected
  line L641 (-98.3551, -74.3118) -> (-98.3551, -73.9118) projected
  line L642 (-98.3551, -73.9118) -> (-97.5651, -73.9118) projected
  line L643 (-97.5651, -73.9118) -> (-97.5651, -74.3118) projected
  line L644 (-95.0251, -75.1118) -> (-95.8151, -75.1118) projected
  line L645 (-95.8151, -75.1118) -> (-95.8151, -74.7118) projected
  line L646 (-95.8151, -74.7118) -> (-95.0251, -74.7118) projected
  line L647 (-95.0251, -74.7118) -> (-95.0251, -75.1118) projected
  line L648 (-97.5651, -75.1118) -> (-98.3551, -75.1118) projected
  line L649 (-98.3551, -75.1118) -> (-98.3551, -74.7118) projected
  line L650 (-98.3551, -74.7118) -> (-97.5651, -74.7118) projected
  line L651 (-97.5651, -74.7118) -> (-97.5651, -75.1118) projected
  line L652 (-114.6451, -68.4618) -> (-116.2451, -68.4618) projected
  line L653 (-116.2451, -68.4618) -> (-116.2451, -67.8118) projected
  line L654 (-116.2451, -67.8118) -> (-114.6451, -67.8118) projected
  line L655 (-114.6451, -67.8118) -> (-114.6451, -68.4618) projected
  line L656 (-114.6451, -76.3618) -> (-116.2451, -76.3618) projected
  line L657 (-116.2451, -76.3618) -> (-116.2451, -75.7118) projected
  line L658 (-116.2451, -75.7118) -> (-114.6451, -75.7118) projected
  line L659 (-114.6451, -75.7118) -> (-114.6451, -76.3618) projected
  line L660 (-113.7801, -69.4868) -> (-114.5701, -69.4868) projected
  line L661 (-114.5701, -69.4868) -> (-114.5701, -69.0868) projected
  line L662 (-114.5701, -69.0868) -> (-113.7801, -69.0868) projected
  line L663 (-113.7801, -69.0868) -> (-113.7801, -69.4868) projected
  line L664 (-116.3201, -69.4868) -> (-117.1101, -69.4868) projected
  line L665 (-117.1101, -69.4868) -> (-117.1101, -69.0868) projected
  line L666 (-117.1101, -69.0868) -> (-116.3201, -69.0868) projected
  line L667 (-116.3201, -69.0868) -> (-116.3201, -69.4868) projected
  line L668 (-113.7801, -70.2868) -> (-114.5701, -70.2868) projected
  line L669 (-114.5701, -70.2868) -> (-114.5701, -69.8868) projected
  line L670 (-114.5701, -69.8868) -> (-113.7801, -69.8868) projected
  line L671 (-113.7801, -69.8868) -> (-113.7801, -70.2868) projected
  line L672 (-116.3201, -70.2868) -> (-117.1101, -70.2868) projected
  line L673 (-117.1101, -70.2868) -> (-117.1101, -69.8868) projected
  line L674 (-117.1101, -69.8868) -> (-116.3201, -69.8868) projected
  line L675 (-116.3201, -69.8868) -> (-116.3201, -70.2868) projected
  line L676 (-113.7801, -71.0868) -> (-114.5701, -71.0868) projected
  line L677 (-114.5701, -71.0868) -> (-114.5701, -70.6868) projected
  line L678 (-114.5701, -70.6868) -> (-113.7801, -70.6868) projected
  line L679 (-113.7801, -70.6868) -> (-113.7801, -71.0868) projected
  line L680 (-116.3201, -71.0868) -> (-117.1101, -71.0868) projected
  line L681 (-117.1101, -71.0868) -> (-117.1101, -70.6868) projected
  line L682 (-117.1101, -70.6868) -> (-116.3201, -70.6868) projected
  line L683 (-116.3201, -70.6868) -> (-116.3201, -71.0868) projected
  line L684 (-113.7801, -71.8868) -> (-114.5701, -71.8868) projected
  line L685 (-114.5701, -71.8868) -> (-114.5701, -71.4868) projected
  line L686 (-114.5701, -71.4868) -> (-113.7801, -71.4868) projected
  line L687 (-113.7801, -71.4868) -> (-113.7801, -71.8868) projected
  line L688 (-116.3201, -71.8868) -> (-117.1101, -71.8868) projected
  line L689 (-117.1101, -71.8868) -> (-117.1101, -71.4868) projected
  line L690 (-117.1101, -71.4868) -> (-116.3201, -71.4868) projected
  line L691 (-116.3201, -71.4868) -> (-116.3201, -71.8868) projected
  line L692 (-113.7801, -72.6868) -> (-114.5701, -72.6868) projected
  line L693 (-114.5701, -72.6868) -> (-114.5701, -72.2868) projected
  line L694 (-114.5701, -72.2868) -> (-113.7801, -72.2868) projected
  line L695 (-113.7801, -72.2868) -> (-113.7801, -72.6868) projected
  line L696 (-116.3201, -72.6868) -> (-117.1101, -72.6868) projected
  line L697 (-117.1101, -72.6868) -> (-117.1101, -72.2868) projected
  line L698 (-117.1101, -72.2868) -> (-116.3201, -72.2868) projected
  line L699 (-116.3201, -72.2868) -> (-116.3201, -72.6868) projected
  line L700 (-113.7801, -73.4868) -> (-114.5701, -73.4868) projected
  line L701 (-114.5701, -73.4868) -> (-114.5701, -73.0868) projected
  line L702 (-114.5701, -73.0868) -> (-113.7801, -73.0868) projected
  line L703 (-113.7801, -73.0868) -> (-113.7801, -73.4868) projected
  line L704 (-116.3201, -73.4868) -> (-117.1101, -73.4868) projected
  line L705 (-117.1101, -73.4868) -> (-117.1101, -73.0868) projected
  line L706 (-117.1101, -73.0868) -> (-116.3201, -73.0868) projected
  line L707 (-116.3201, -73.0868) -> (-116.3201, -73.4868) projected
  line L708 (-113.7801, -74.2868) -> (-114.5701, -74.2868) projected
  line L709 (-114.5701, -74.2868) -> (-114.5701, -73.8868) projected
  line L710 (-114.5701, -73.8868) -> (-113.7801, -73.8868) projected
  line L711 (-113.7801, -73.8868) -> (-113.7801, -74.2868) projected
  line L712 (-116.3201, -74.2868) -> (-117.1101, -74.2868) projected
  line L713 (-117.1101, -74.2868) -> (-117.1101, -73.8868) projected
  line L714 (-117.1101, -73.8868) -> (-116.3201, -73.8868) projected
  line L715 (-116.3201, -73.8868) -> (-116.3201, -74.2868) projected
  line L716 (-113.7801, -75.0868) -> (-114.5701, -75.0868) projected
  line L717 (-114.5701, -75.0868) -> (-114.5701, -74.6868) projected
  line L718 (-114.5701, -74.6868) -> (-113.7801, -74.6868) projected
  line L719 (-113.7801, -74.6868) -> (-113.7801, -75.0868) projected
  line L720 (-116.3201, -75.0868) -> (-117.1101, -75.0868) projected
  line L721 (-117.1101, -75.0868) -> (-117.1101, -74.6868) projected
  line L722 (-117.1101, -74.6868) -> (-116.3201, -74.6868) projected
  line L723 (-116.3201, -74.6868) -> (-116.3201, -75.0868) projected
  line L724 (-39.4576, -30.7368) -> (-41.0576, -30.7368) projected
  line L725 (-41.0576, -30.7368) -> (-41.0576, -30.0868) projected
  line L726 (-41.0576, -30.0868) -> (-39.4576, -30.0868) projected
  line L727 (-39.4576, -30.0868) -> (-39.4576, -30.7368) projected
  line L728 (-39.4576, -38.6368) -> (-41.0576, -38.6368) projected
  line L729 (-41.0576, -38.6368) -> (-41.0576, -37.9868) projected
  line L730 (-41.0576, -37.9868) -> (-39.4576, -37.9868) projected
  line L731 (-39.4576, -37.9868) -> (-39.4576, -38.6368) projected
  line L732 (-38.5926, -31.7618) -> (-39.3826, -31.7618) projected
  line L733 (-39.3826, -31.7618) -> (-39.3826, -31.3618) projected
  line L734 (-39.3826, -31.3618) -> (-38.5926, -31.3618) projected
  line L735 (-38.5926, -31.3618) -> (-38.5926, -31.7618) projected
  line L736 (-41.1326, -31.7618) -> (-41.9226, -31.7618) projected
  line L737 (-41.9226, -31.7618) -> (-41.9226, -31.3618) projected
  line L738 (-41.9226, -31.3618) -> (-41.1326, -31.3618) projected
  line L739 (-41.1326, -31.3618) -> (-41.1326, -31.7618) projected
  line L740 (-38.5926, -32.5618) -> (-39.3826, -32.5618) projected
  line L741 (-39.3826, -32.5618) -> (-39.3826, -32.1618) projected
  line L742 (-39.3826, -32.1618) -> (-38.5926, -32.1618) projected
  line L743 (-38.5926, -32.1618) -> (-38.5926, -32.5618) projected
  line L744 (-41.1326, -32.5618) -> (-41.9226, -32.5618) projected
  line L745 (-41.9226, -32.5618) -> (-41.9226, -32.1618) projected
  line L746 (-41.9226, -32.1618) -> (-41.1326, -32.1618) projected
  line L747 (-41.1326, -32.1618) -> (-41.1326, -32.5618) projected
  line L748 (-38.5926, -33.3618) -> (-39.3826, -33.3618) projected
  line L749 (-39.3826, -33.3618) -> (-39.3826, -32.9618) projected
  line L750 (-39.3826, -32.9618) -> (-38.5926, -32.9618) projected
  line L751 (-38.5926, -32.9618) -> (-38.5926, -33.3618) projected
  line L752 (-41.1326, -33.3618) -> (-41.9226, -33.3618) projected
  line L753 (-41.9226, -33.3618) -> (-41.9226, -32.9618) projected
  line L754 (-41.9226, -32.9618) -> (-41.1326, -32.9618) projected
  line L755 (-41.1326, -32.9618) -> (-41.1326, -33.3618) projected
  line L756 (-38.5926, -34.1618) -> (-39.3826, -34.1618) projected
  line L757 (-39.3826, -34.1618) -> (-39.3826, -33.7618) projected
  line L758 (-39.3826, -33.7618) -> (-38.5926, -33.7618) projected
  line L759 (-38.5926, -33.7618) -> (-38.5926, -34.1618) projected
  line L760 (-41.1326, -34.1618) -> (-41.9226, -34.1618) projected
  line L761 (-41.9226, -34.1618) -> (-41.9226, -33.7618) projected
  line L762 (-41.9226, -33.7618) -> (-41.1326, -33.7618) projected
  line L763 (-41.1326, -33.7618) -> (-41.1326, -34.1618) projected
  line L764 (-38.5926, -34.9618) -> (-39.3826, -34.9618) projected
  line L765 (-39.3826, -34.9618) -> (-39.3826, -34.5618) projected
  line L766 (-39.3826, -34.5618) -> (-38.5926, -34.5618) projected
  line L767 (-38.5926, -34.5618) -> (-38.5926, -34.9618) projected
  line L768 (-41.1326, -34.9618) -> (-41.9226, -34.9618) projected
  line L769 (-41.9226, -34.9618) -> (-41.9226, -34.5618) projected
  line L770 (-41.9226, -34.5618) -> (-41.1326, -34.5618) projected
  line L771 (-41.1326, -34.5618) -> (-41.1326, -34.9618) projected
  line L772 (-38.5926, -35.7618) -> (-39.3826, -35.7618) projected
  line L773 (-39.3826, -35.7618) -> (-39.3826, -35.3618) projected
  line L774 (-39.3826, -35.3618) -> (-38.5926, -35.3618) projected
  line L775 (-38.5926, -35.3618) -> (-38.5926, -35.7618) projected
  line L776 (-41.1326, -35.7618) -> (-41.9226, -35.7618) projected
  line L777 (-41.9226, -35.7618) -> (-41.9226, -35.3618) projected
  line L778 (-41.9226, -35.3618) -> (-41.1326, -35.3618) projected
  line L779 (-41.1326, -35.3618) -> (-41.1326, -35.7618) projected
  line L780 (-38.5926, -36.5618) -> (-39.3826, -36.5618) projected
  line L781 (-39.3826, -36.5618) -> (-39.3826, -36.1618) projected
  line L782 (-39.3826, -36.1618) -> (-38.5926, -36.1618) projected
  line L783 (-38.5926, -36.1618) -> (-38.5926, -36.5618) projected
  line L784 (-41.1326, -36.5618) -> (-41.9226, -36.5618) projected
  line L785 (-41.9226, -36.5618) -> (-41.9226, -36.1618) projected
  line L786 (-41.9226, -36.1618) -> (-41.1326, -36.1618) projected
  line L787 (-41.1326, -36.1618) -> (-41.1326, -36.5618) projected
  line L788 (-38.5926, -37.3618) -> (-39.3826, -37.3618) projected
  line L789 (-39.3826, -37.3618) -> (-39.3826, -36.9618) projected
  line L790 (-39.3826, -36.9618) -> (-38.5926, -36.9618) projected
  line L791 (-38.5926, -36.9618) -> (-38.5926, -37.3618) projected
  line L792 (-41.1326, -37.3618) -> (-41.9226, -37.3618) projected
  line L793 (-41.9226, -37.3618) -> (-41.9226, -36.9618) projected
  line L794 (-41.9226, -36.9618) -> (-41.1326, -36.9618) projected
  line L795 (-41.1326, -36.9618) -> (-41.1326, -37.3618) projected
  line L796 (-78.6251, -19.4368) -> (-77.0251, -19.4368) projected
  line L797 (-77.0251, -19.4368) -> (-77.0251, -20.0868) projected
  line L798 (-77.0251, -20.0868) -> (-78.6251, -20.0868) projected
  line L799 (-78.6251, -20.0868) -> (-78.6251, -19.4368) projected
  line L800 (-78.6251, -11.5368) -> (-77.0251, -11.5368) projected
  line L801 (-77.0251, -11.5368) -> (-77.0251, -12.1868) projected
  line L802 (-77.0251, -12.1868) -> (-78.6251, -12.1868) projected
  line L803 (-78.6251, -12.1868) -> (-78.6251, -11.5368) projected
  line L804 (-79.4901, -18.4118) -> (-78.7001, -18.4118) projected
  line L805 (-78.7001, -18.4118) -> (-78.7001, -18.8118) projected
  line L806 (-78.7001, -18.8118) -> (-79.4901, -18.8118) projected
  line L807 (-79.4901, -18.8118) -> (-79.4901, -18.4118) projected
  line L808 (-76.9501, -18.4118) -> (-76.1601, -18.4118) projected
  line L809 (-76.1601, -18.4118) -> (-76.1601, -18.8118) projected
  line L810 (-76.1601, -18.8118) -> (-76.9501, -18.8118) projected
  line L811 (-76.9501, -18.8118) -> (-76.9501, -18.4118) projected
  line L812 (-79.4901, -17.6118) -> (-78.7001, -17.6118) projected
  line L813 (-78.7001, -17.6118) -> (-78.7001, -18.0118) projected
  line L814 (-78.7001, -18.0118) -> (-79.4901, -18.0118) projected
  line L815 (-79.4901, -18.0118) -> (-79.4901, -17.6118) projected
  line L816 (-76.9501, -17.6118) -> (-76.1601, -17.6118) projected
  line L817 (-76.1601, -17.6118) -> (-76.1601, -18.0118) projected
  line L818 (-76.1601, -18.0118) -> (-76.9501, -18.0118) projected
  line L819 (-76.9501, -18.0118) -> (-76.9501, -17.6118) projected
  line L820 (-79.4901, -16.8118) -> (-78.7001, -16.8118) projected
  line L821 (-78.7001, -16.8118) -> (-78.7001, -17.2118) projected
  line L822 (-78.7001, -17.2118) -> (-79.4901, -17.2118) projected
  line L823 (-79.4901, -17.2118) -> (-79.4901, -16.8118) projected
  line L824 (-76.9501, -16.8118) -> (-76.1601, -16.8118) projected
  line L825 (-76.1601, -16.8118) -> (-76.1601, -17.2118) projected
  line L826 (-76.1601, -17.2118) -> (-76.9501, -17.2118) projected
  line L827 (-76.9501, -17.2118) -> (-76.9501, -16.8118) projected
  line L828 (-79.4901, -16.0118) -> (-78.7001, -16.0118) projected
  line L829 (-78.7001, -16.0118) -> (-78.7001, -16.4118) projected
  line L830 (-78.7001, -16.4118) -> (-79.4901, -16.4118) projected
  line L831 (-79.4901, -16.4118) -> (-79.4901, -16.0118) projected
  line L832 (-76.9501, -16.0118) -> (-76.1601, -16.0118) projected
  line L833 (-76.1601, -16.0118) -> (-76.1601, -16.4118) projected
  line L834 (-76.1601, -16.4118) -> (-76.9501, -16.4118) projected
  line L835 (-76.9501, -16.4118) -> (-76.9501, -16.0118) projected
  line L836 (-79.4901, -15.2118) -> (-78.7001, -15.2118) projected
  line L837 (-78.7001, -15.2118) -> (-78.7001, -15.6118) projected
  line L838 (-78.7001, -15.6118) -> (-79.4901, -15.6118) projected
  line L839 (-79.4901, -15.6118) -> (-79.4901, -15.2118) projected
  line L840 (-76.9501, -15.2118) -> (-76.1601, -15.2118) projected
  line L841 (-76.1601, -15.2118) -> (-76.1601, -15.6118) projected
  line L842 (-76.1601, -15.6118) -> (-76.9501, -15.6118) projected
  line L843 (-76.9501, -15.6118) -> (-76.9501, -15.2118) projected
  line L844 (-79.4901, -14.4118) -> (-78.7001, -14.4118) projected
  line L845 (-78.7001, -14.4118) -> (-78.7001, -14.8118) projected
  line L846 (-78.7001, -14.8118) -> (-79.4901, -14.8118) projected
  line L847 (-79.4901, -14.8118) -> (-79.4901, -14.4118) projected
  line L848 (-76.9501, -14.4118) -> (-76.1601, -14.4118) projected
  line L849 (-76.1601, -14.4118) -> (-76.1601, -14.8118) projected
  line L850 (-76.1601, -14.8118) -> (-76.9501, -14.8118) projected
  line L851 (-76.9501, -14.8118) -> (-76.9501, -14.4118) projected
  line L852 (-79.4901, -13.6118) -> (-78.7001, -13.6118) projected
  line L853 (-78.7001, -13.6118) -> (-78.7001, -14.0118) projected
  line L854 (-78.7001, -14.0118) -> (-79.4901, -14.0118) projected
  line L855 (-79.4901, -14.0118) -> (-79.4901, -13.6118) projected
  line L856 (-76.9501, -13.6118) -> (-76.1601, -13.6118) projected
  line L857 (-76.1601, -13.6118) -> (-76.1601, -14.0118) projected
  line L858 (-76.1601, -14.0118) -> (-76.9501, -14.0118) projected
  line L859 (-76.9501, -14.0118) -> (-76.9501, -13.6118) projected
  line L860 (-79.4901, -12.8118) -> (-78.7001, -12.8118) projected
  line L861 (-78.7001, -12.8118) -> (-78.7001, -13.2118) projected
  line L862 (-78.7001, -13.2118) -> (-79.4901, -13.2118) projected
  line L863 (-79.4901, -13.2118) -> (-79.4901, -12.8118) projected
  line L864 (-76.9501, -12.8118) -> (-76.1601, -12.8118) projected
  line L865 (-76.1601, -12.8118) -> (-76.1601, -13.2118) projected
  line L866 (-76.1601, -13.2118) -> (-76.9501, -13.2118) projected
  line L867 (-76.9501, -13.2118) -> (-76.9501, -12.8118) projected
  line L868 (-97.2926, -57.0118) -> (-95.6926, -57.0118) projected
  line L869 (-95.6926, -57.0118) -> (-95.6926, -57.6618) projected
  line L870 (-95.6926, -57.6618) -> (-97.2926, -57.6618) projected